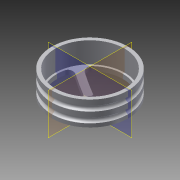
# Autodesk Inventor part: Rueda1
Saved by Autodesk Inventor 2013 (Build 170138000, 138)
## iProperties
Created: 2012-12-03
Part Number: Rueda1
Material: ABS Plastic
Document SubType Name: Modeling
Designer: ALUMNO
Density: 1 g/cm^3
Author: ALUMNO
Autodesk Inventor part; units mm, degrees
ref_plane "XY Plane" through (0, 0, 0) normal (0, 0, 1) x (1, 0, 0)
sketch "Sketch1" plane through (0, 0, 0) normal (0, 0, 1) x (1, 0, 0)
  line L0 (-19.5, 0) -> (19.5, 0) construction
  line L1 (-1.4361, -1) -> (1.4361, -1)
  line L2 (0, -3.25) -> (0, -10.5) construction
  line L3 (0, 31.6864) -> (0, -32.6182) construction
  line L4 (2, -2.5617) -> (2, -19.3972)
  line L5 (-2, -2.5617) -> (-2, -19.3972)
  line L6 (2.8146, 1.625) -> (9.0933, 5.25) construction
  line L7 (-2.8146, 1.625) -> (-9.0933, 5.25) construction
  line L8 (3.2185, -0.4512) -> (17.7984, 7.9665)
  line L9 (1.2185, 3.0129) -> (15.7984, 11.4306)
  arc A0 (2, -19.3972) -> (17.7984, 7.9665) centre (0, 0) ccw
  line L10 (-15.7984, 11.4306) -> (-1.2185, 3.0129)
  line L11 (-17.7984, 7.9665) -> (-3.2185, -0.4512)
  arc A1 (15.7984, 11.4306) -> (-15.7984, 11.4306) centre (0, 0) ccw
  arc A2 (-17.7984, 7.9665) -> (-2, -19.3972) centre (0, 0) ccw
  arc A3 (-3.2185, -0.4512) -> (-2, -2.5617) centre (0, 0) ccw
  arc A4 (2, -2.5617) -> (3.2185, -0.4512) centre (0, 0) ccw
  line L12 (0, 0) -> (2.6981, 7.4129) construction
  line L13 (0, 0) -> (-2.481, 6.8165) construction
  line L14 (0.5985, 1.6445) -> (1.1116, 3.054)
  line L15 (-0.5985, 1.6445) -> (-1.1116, 3.054)
  arc A5 (1.2185, 3.0129) -> (1.1116, 3.054) centre (0, 0) ccw
  arc A6 (-1.1116, 3.054) -> (-1.2185, 3.0129) centre (0, 0) ccw
  arc A7 (1.4361, -1) -> (0.5985, 1.6445) centre (0, 0) ccw
  arc A8 (-0.5985, 1.6445) -> (-1.4361, -1) centre (0, 0) ccw
  circle A9 centre (0, 0) radius 22.5
  dimension "d3" = 1
  dimension "d4" = 2
  dimension "d5" = 2
  dimension "d8" = 360
  dimension "d10" = 2
  dimension "d11" = 2
  dimension "d12" = 2
  dimension "d13" = 2
  dimension "d17" = 3.25
  dimension "d18" = 3.25
  dimension "d19" = 20
  dimension "d20" = 20
  dimension "d21" = 3.25
  dimension "d22" = 3.25
  dimension "d23" = 1.75
  dimension "d24" = 1.75
  dimension "d25" = 45
  dimension "d81" = 3
  dimension "d84" = 3
  dimension "d85" = 3
  constraints: 30 end point, 21 point on circle, 10 centre point, 7 parallel, 5 point on line, 4 coincident, 1 collinear, 1 horizontal, 1 midpoint, 1 perpendicular, 10 other
  measures "d3" distance between parallel lines of L1 L0
  measures "d4" distance between parallel lines of L4 L2
  measures "d5" distance between parallel lines of L2 L5
  measures "d10" distance between parallel lines of L9 L6
  measures "d11" distance between parallel lines of L8 L6
  measures "d12" distance between parallel lines of L10 L7
  measures "d13" distance between parallel lines of L7 L11
  measures "d17" radius of A4
  measures "d18" radius of A3
  measures "d19" angle of L3 L12
  measures "d20" angle of L3 L13
  measures "d21" radius of A5
  measures "d22" radius of A6
  measures "d23" radius of A8
  measures "d24" radius of A7
  measures "d25" diameter of A9
  measures "d81" radial gap between concentric circles of A9 A1
  measures "d84" radial gap between concentric circles of A0 A9
  measures "d85" radial gap between concentric circles of A9 A2
extrude "Extrusion1" add sketch "Sketch1" along normal blind 16
fillet "Fillet10" radius 1 6 edges at (3.2185, -0.4512, 8) (2, -2.5617, 8) (-3.2185, -0.4512, 8) (-2, -2.5617, 8) (-1.2185, 3.0129, 8) (1.2185, 3.0129, 8)
fillet "Fillet11" radius 3 6 edges at (-17.7984, 7.9665, 8) (-15.7984, 11.4306, 8) (15.7984, 11.4306, 8) (17.7984, 7.9665, 8) (2, -19.3972, 8) (-2, -19.3972, 8)
sketch "Sketch5" plane through (0, 0, 16) normal (0, 0, 1) x (1, 0, 0)
  arc A0 (-19.048, 4.1741) -> (-5.9091, -18.5831) centre (0, 0) ccw projected
  circle A1 centre (0, 0) radius 22.5 projected
  circle A2 centre (0, 0) radius 22.5
  circle A3 centre (0, 0) radius 19.5
  constraints: 2 centre point, 2 coincident, 2 concentric
extrude "Extrusion2" add sketch "Sketch5" along normal blind 6
sketch "Sketch4" plane through (0, 0, 0) normal (0, 1, 0) x (-1, 0, 0)
  line L0 (0, 7.6708) -> (0, -6.5685) construction
  line L1 (22.4394, 8.3109) -> (22.4394, 10.67) construction
  line L2 (22.4394, 10.67) -> (22.4394, 8.3109) construction
  line L3 (22.4394, 8.3109) -> (22.4394, 11.3109) construction
  circle A0 centre (22.4394, 11.3109) radius 1.5
  line L4 (22.4394, 16.67) -> (22.4394, 14.3109) construction
  circle A1 centre (22.4394, 17.3109) radius 1.5
  point P0 (0, 0)
  dimension "d104" = 3
  dimension "d105" = 3
  dimension "d108" = 6
  constraints: 10 end point, 2 centre point, 2 coincident, 2 collinear, 2 point on line, 2 vertical, 1 parallel, 5 other
  measures "d104" distance of L1.start L3.end
  measures "d105" diameter of A0
  measures "d108" distance of L1.end L4.start
revolve "Revolution2" cut sketch "Sketch4" angle 360 about axis through (0, 0, 7.6708) along (0, 0, -1)
sketch "Sketch6" plane through (0, 0, 0) normal (0, 1, 0) x (-1, 0, 0)
  line L0 (9.8861, 4.3803) -> (14.8355, 5.5652)
  line L1 (14.8355, 5.5652) -> (25.5714, 8.5321)
  line L2 (25.5714, 8.5321) -> (25.5714, -1.6223)
  line L3 (25.5714, -1.6223) -> (6.1145, -1.6223)
  line L4 (0, -3.6531) -> (0, 10.563) projected
  line L5 (-0.0074, -1.329) -> (-0.0074, -1.6223)
  line L6 (-0.0074, -1.6223) -> (0, -1.6223)
  line L7 (5.9046, -1.6223) -> (2.6812, -1.6223)
  line L8 (5.9046, -1.6223) -> (6.1145, -1.6223)
  line L9 (2.6812, -1.6223) -> (2.6812, 0.6149)
  line L10 (2.6812, 0.6149) -> (3.8167, 4.3803)
  line L11 (3.8167, 4.3803) -> (9.8861, 4.3803)
  point P0 (0, 0)
  point P1 (0, 2.0136)
  constraints: 22 end point, 4 perpendicular, 2 point on line, 1 collinear, 1 parallel
revolve "Revolution3" cut sketch "Sketch6" angle 360 about axis through (0, 0, -10) along (0, 0, 1)
sketch "Sketch7" plane through (0, 0, 0) normal (1, 0, 0) x (0, 1, 0)
  line L0 (-20.4584, 28.0794) -> (-20.4584, 9.657)
  line L1 (-20.4584, 9.657) -> (-20.2457, 9.657)
  line L2 (-4.1823, 28.0794) -> (-20.4584, 28.0794)
  line L3 (0, -5.6159) -> (0, 33.6953) projected
  line L4 (-4.1823, 28.0794) -> (0, 28.0794)
  line L5 (-2.1367, 6.743) -> (-3.35, 6.743)
  line L6 (-2.1367, 6.743) -> (-2.1367, 6.7329)
  line L7 (-2.1367, 6.7329) -> (0, 6.7329)
  line L8 (-20.2457, 9.657) -> (-9.8094, 7.3602)
  line L9 (-9.8094, 7.3602) -> (-3.35, 6.743)
  point P0 (0, 0)
  point P1 (0, 6.743)
  constraints: 18 end point, 4 perpendicular, 3 point on line, 2 parallel, 1 vertical
revolve "Revolution4" cut sketch "Sketch7" angle 360 about axis through (0, 0, -10) along (0, 0, 1)
equation "\"d5\" = d4"
equation "\"d11\" = d10"
equation "\"d12\" = d10"
equation "\"d13\" = d10"
equation "\"d18\" = d17"
equation "\"d20\" = d19"
equation "\"d21\" = d17"
equation "\"d22\" = d17"
equation "\"d24\" = d23"
body "Solid1"
